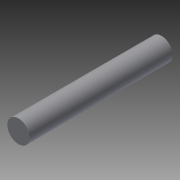
# Autodesk Inventor part: Part76
Saved by Autodesk Inventor 2015 (Build 190159000, 159)
## iProperties
Created: 2015-01-11
Part Number: Part76
Material: Generic
Document SubType Name: Modeling
Designer: mastkee16
Density: 1 g/cm^3
Appearance: Default
Author: mastkee16
Autodesk Inventor part; units mm, degrees
ref_plane "YZ Plane" through (0, 0, 0) normal (1, 0, 0) x (0, 1, 0)
ref_plane "XZ Plane" through (0, 0, 0) normal (0, 1, 0) x (-1, 0, 0)
ref_plane "XY Plane" through (0, 0, 0) normal (0, 0, 1) x (1, 0, 0)
sketch "Sketch1" plane through (0, 0, 0) normal (0, 0, 1) x (1, 0, 0)
  circle A0 centre (2.662, 2.3292) radius 3.9687
  point P0 (0, 0)
  dimension "d0" = 7.9375
  dimension "d0" = 7.9375
  constraints: 1 centre point
  measures "d0" diameter of A0
extrude "Extrusion1" add sketch "Sketch1" along normal blind 50.8
body "Solid1"
